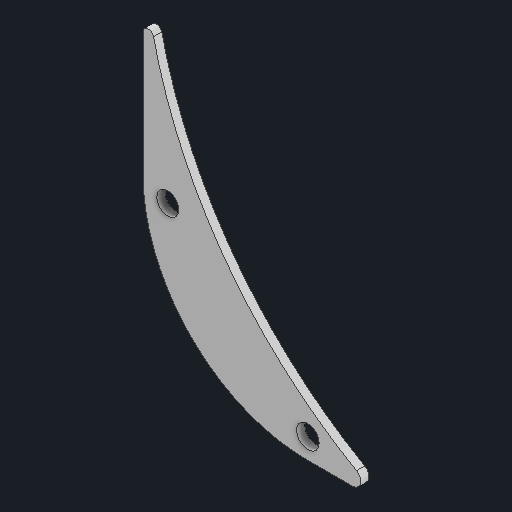
# Autodesk Inventor part: ramp_v2
Saved by Autodesk Inventor 2025 (Build 290162000, 162)
## iProperties
Created: 2024-10-12
Part Number: ramp_v2
Material: Generic
Document SubType Name: Modeling
Designer: Averey Ku
Density: 1 g/cm^3
Appearance: Default
Author: Averey Ku
Autodesk Inventor part; units mm, degrees
ref_plane "YZ Plane" through (0, 0, 0) normal (1, 0, 0) x (0, 1, 0)
ref_plane "XZ Plane" through (0, 0, 0) normal (0, 1, 0) x (-1, 0, 0)
ref_plane "XY Plane" through (0, 0, 0) normal (0, 0, 1) x (1, 0, 0)
sketch "Sketch1" plane through (0, 0, 0) normal (0, 0, 1) x (1, 0, 0)
  circle A0 centre (-5.4749, -29.1324) radius 2.1844
  arc A1 (-35.2179, 22.7309) -> (3.9033, -30.1393) centre (44.3765, 40.7176) ccw
  line L0 (-37.2249, 22.5069) -> (-37.2249, -1.3553)
  arc A2 (-35.2179, 22.7309) -> (-37.2249, 22.5069) centre (-36.2089, 22.5069) ccw
  line L1 (3.1159, -33.1053) -> (-5.4749, -33.1053)
  arc A3 (3.1159, -33.1053) -> (3.9033, -30.1393) centre (3.1159, -31.5178) ccw
  arc A4 (-37.2249, -1.3553) -> (-5.4749, -33.1053) centre (-5.4749, -1.3553) ccw
  circle A5 centre (-32.4624, -3.7324) radius 2.1209
  point P0 (0, 0)
  point P1 (-37.2249, 40.7176)
  point P2 (9.6063, -33.1053)
  dimension "d0" = 1.016
  dimension "d1" = 1.5875
  dimension "d2" = 31.75
  constraints: 10 point on circle, 7 tangent, 6 centre point, 4 end point, 2 point on line, 2 vertical, 1 perpendicular, 1 other
  measures "d0" radius of A2
  measures "d1" radius of A3
  measures "d2" radius of A4
extrude "Extrusion1" add sketch "Sketch1" along normal blind 1.5875
body "Solid1"
